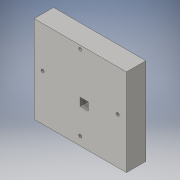
# Autodesk Inventor part: speakerback
Saved by Autodesk Inventor 2016 (Build 200138000, 138)
## iProperties
Created: 2018-09-28
Part Number: speakerback
Material: Generic
Document SubType Name: Modeling
Designer: student
Density: 1 g/cm^3
Appearance: Default
Author: student
Autodesk Inventor part; units mm, degrees
ref_plane "YZ Plane" through (0, 0, 0) normal (1, 0, 0) x (0, 1, 0)
ref_plane "XZ Plane" through (0, 0, 0) normal (0, 1, 0) x (-1, 0, 0)
ref_plane "XY Plane" through (0, 0, 0) normal (0, 0, 1) x (1, 0, 0)
sketch "Sketch1" plane through (0, 0, 0) normal (0, 0, 1) x (1, 0, 0)
  line L0 (0, 0) -> (120.65, 0)
  line L1 (120.65, 0) -> (120.65, 113.9317)
  line L2 (0, 113.9317) -> (0, 0)
  circle A0 centre (11.2141, 60.325) radius 1.9431
  circle A1 centre (60.325, 11.2141) radius 1.9431
  circle A2 centre (109.4359, 60.325) radius 1.9431
  circle A3 centre (60.325, 109.4359) radius 1.9431
  line L3 (60.071, 55.0418) -> (70.739, 55.0418)
  line L4 (70.739, 44.8818) -> (60.071, 44.8818)
  line L5 (60.071, 55.0418) -> (60.071, 44.8818)
  line L6 (70.739, 55.0418) -> (70.739, 44.8818)
  line L7 (60.325, 113.9317) -> (120.65, 113.9317)
  line L8 (60.325, 113.9317) -> (0, 113.9317)
  point P0 (60.325, 60.325)
  dimension "d10" = 3.8862
  dimension "d13" = 360
  dimension "d44" = 4.4958
  constraints: 18 end point, 4 centre point, 2 perpendicular, 2 vertical, 1 horizontal, 1 parallel, 1 point on line, 9 other
  measures "d10" diameter of A0
  measures "d44" distance of A3.centre L7.start
extrude "Extrusion6" add sketch "Sketch1" along normal blind 25.4
body "Solid6"
